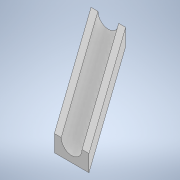
# Autodesk Inventor part: Ramp Main
Saved by Autodesk Inventor 2021 (Build 250183000, 183)
## iProperties
Created: 2021-04-12
Part Number: Ramp Main
Material: Generic
Document SubType Name: Modeling
Designer: Nabeel Azafer
Density: 1 g/cm^3
Appearance: Default
Author: Nabeel Azafer
Autodesk Inventor part; units mm, degrees
ref_plane "YZ Plane" through (0, 0, 0) normal (1, 0, 0) x (0, 1, 0)
ref_plane "XZ Plane" through (0, 0, 0) normal (0, 1, 0) x (-1, 0, 0)
sketch "Sketch2" plane through (0, 0, 0) normal (0, 0, 1) x (1, 0, 0)
  line L0 (0, 0) -> (25, 0)
  line L1 (25, 0) -> (25, 12)
  line L2 (0, 12) -> (0, 0)
  line L3 (0, 12) -> (5, 12)
  line L4 (25, 12) -> (20, 12)
  arc A0 (5, 12) -> (20, 12) centre (12.5, 12) ccw
  dimension "d1" = 25
  dimension "d2" = 12
  dimension "d3" = 5
  dimension "d4" = 5
  dimension "d5" = 7.5
  constraints: 10 end point, 3 horizontal, 2 point on circle, 1 centre point, 1 parallel, 1 perpendicular
  measures "d1" distance of L1.end L2.start
  measures "d2" distance of L2.start L0.start
  measures "d3" distance of L2.start L3.end
  measures "d4" distance of L1.end L4.end
  measures "d5" radius of A0
ref_plane "Work Plane1" through (0, 0, 54.5) normal (0, 0, 1) x (1, 0, 0)
sketch "Sketch3" plane through (0, 0, 54.5) normal (0, 0, 1) x (1, 0, 0)
  line L0 (28, -25.729) -> (33, -25.729)
  line L1 (28, -25.729) -> (28, -37.729)
  line L2 (28, -37.729) -> (53, -37.729)
  line L3 (53, -37.729) -> (53, -25.729)
  line L4 (53, -25.729) -> (48, -25.729)
  arc A0 (33, -25.729) -> (48, -25.729) centre (40.5, -25.729) ccw
  point P0 (0, 0)
  dimension "d15" = 5
  dimension "d17" = 25
  dimension "d19" = 5
  dimension "d22" = 7.5
  dimension "d28" = 12
  constraints: 10 end point, 3 perpendicular, 2 point on circle, 1 centre point, 1 horizontal, 1 vertical
  measures "d15" distance of L0.start L0.end
  measures "d17" distance of L1.end L2.end
  measures "d19" distance of L3.end L4.end
  measures "d22" radius of A0
  measures "d28" distance of L0.start L1.end
loft "Loft1" add profiles "Sketch2", "Sketch3"
sketch "Sketch4" plane through (0, 0, 0) normal (-0.8895, 0, 0.457) x (0.457, 0, 0.8895)
  point P0 (0, 0)
body "Solid1"
